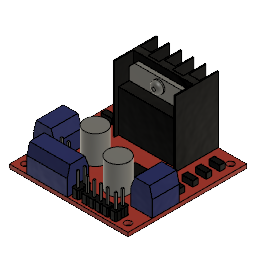
L298n H-Bridge (Autodesk Fusion 360 design; units mm, degrees)
Autodesk Fusion 360 part; units mm, degrees
note: some values were not read from the file. Chosen so that the rebuilt part matches the saved one: which bodies a step acts on; which face or edge a step refers to. Set by a fixed rule: which sketch regions a step uses.
sketch "Sketch1" plane through (0, 0, 0) normal (0, 0, 1) x (1, 0, 0)
  line L0 (0, 0) -> (-70, 0) construction
  line L1 (22, 22) -> (22, -22)
  line L2 (22, -22) -> (-22, -22)
  line L3 (-22, -22) -> (-22, 22)
  line L4 (22, -13) -> (-22, -13) construction
  line L5 (-22, -14) -> (22, -14) construction
  line L6 (-15.5, -22) -> (-15.5, -14) construction
  line L7 (-15.5, -22) -> (-0.5, -22)
  line L8 (-0.5, -22) -> (-0.5, -14)
  line L9 (-0.5, -14) -> (-15.5, -14)
  line L10 (-15.5, -14) -> (-15.5, -22)
  line L11 (-22, -13) -> (-14, -13)
  line L12 (-14, -13) -> (-14, -3)
  line L13 (-14, -3) -> (-22, -3)
  line L14 (-22, -3) -> (-22, -13)
  line L15 (22, -13) -> (14, -13)
  line L16 (14, -13) -> (14, -3)
  line L17 (14, -3) -> (22, -3)
  line L18 (22, -3) -> (22, -13)
  line L19 (-12, 22) -> (-12, 0) construction
  line L20 (12, 22) -> (12, 0) construction
  line L21 (11, 22) -> (11.5, 22)
  line L22 (0, 22) -> (-11.5, 22)
  line L23 (-11.5, 22) -> (-11.5, 6)
  line L24 (11.5, 6) -> (11.5, 22)
  line L25 (-11.5, 22) -> (-11.5, 6)
  line L26 (0, -22) -> (2.5, -22) construction
  line L27 (0, -22) -> (0, -21) construction
  line L28 (0.5, -21) -> (2, -21)
  line L29 (2.5, -18) -> (2.5, -16.5)
  line L30 (2, -16) -> (0.5, -16)
  line L31 (0, -19) -> (0, -20.5)
  line L32 (2.5, -21) -> (3.5, -21) construction
  line L33 (4, -21) -> (5.5388, -21)
  line L34 (13.5, -20.5) -> (13.5, -18.9999)
  line L35 (7.9986, -18.5) -> (6.5388, -18.5)
  line L36 (3.5, -19) -> (3.5, -20.5)
  line L37 (13.5, -21) -> (14, -21) construction
  line L38 (14.5, -21) -> (16, -21)
  line L39 (16.5, -18) -> (16.5, -16.5)
  line L40 (16, -16) -> (14.5, -16)
  line L41 (14, -19) -> (14, -20.5)
  line L42 (-14, -14) -> (-14, -13.5) construction
  line L43 (-14, -13.5) -> (-13.5, -13.5) construction
  line L44 (-10.5, -13.5) -> (-9, -13.5)
  line L45 (-8.5, -13) -> (-8.5, -11.5)
  line L46 (-11.5, -11) -> (-13, -11)
  line L47 (-13.5, -11.5) -> (-13.5, -13)
  line L48 (1.25, -21) -> (1.25, -16) construction
  line L49 (0.5, -18.5) -> (2, -18.5)
  line L50 (3.5, -19.75) -> (13.5, -19.75) construction
  line L51 (8.4986, -19) -> (8.4986, -20.5)
  line L52 (4, -18.5) -> (5.5388, -18.5)
  line L53 (6.0388, -19) -> (6.0388, -20.5)
  line L54 (8.9986, -18.5) -> (10.5014, -18.5)
  line L55 (11.0014, -18.9999) -> (11.0014, -20.5)
  line L56 (14.5, -18.5) -> (16, -18.5)
  arc A0 (0.5, -18.5) -> (0, -19) centre (0.5, -19) ccw
  line L57 (0, -16.5) -> (0, -18)
  arc A1 (0, -18) -> (0.5, -18.5) centre (0.5, -18) ccw
  arc A2 (2, -18.5) -> (2.5, -18) centre (2, -18) ccw
  line L58 (2.5, -20.5) -> (2.5, -19)
  arc A3 (2.5, -19) -> (2, -18.5) centre (2, -19) ccw
  arc A4 (0.5, -16) -> (0, -16.5) centre (0.5, -16.5) ccw
  arc A5 (2.5, -16.5) -> (2, -16) centre (2, -16.5) ccw
  arc A6 (0, -20.5) -> (0.5, -21) centre (0.5, -20.5) ccw
  arc A7 (2, -21) -> (2.5, -20.5) centre (2, -20.5) ccw
  arc A8 (6.5388, -18.5) -> (6.0388, -19) centre (6.5388, -19) ccw
  arc A9 (5.5388, -21) -> (6.0388, -20.5) centre (5.5388, -20.5) ccw
  line L59 (6.5388, -21) -> (7.9986, -21)
  line L60 (8.9986, -21) -> (10.5014, -21)
  line L61 (11.5014, -21) -> (13, -21)
  arc A10 (6.0388, -20.5) -> (6.5388, -21) centre (6.5388, -20.5) ccw
  arc A11 (8.4986, -19) -> (7.9986, -18.5) centre (7.9986, -19) ccw
  arc A12 (7.9986, -21) -> (8.4986, -20.5) centre (7.9986, -20.5) ccw
  arc A13 (3.5, -20.5) -> (4, -21) centre (4, -20.5) ccw
  arc A14 (4, -18.5) -> (3.5, -19) centre (4, -19) ccw
  arc A15 (8.9986, -18.5) -> (8.4986, -19) centre (8.9986, -19) ccw
  arc A16 (8.4986, -20.5) -> (8.9986, -21) centre (8.9986, -20.5) ccw
  arc A17 (11.0014, -19) -> (10.5014, -18.5) centre (10.5014, -19) ccw
  arc A18 (10.5014, -21) -> (11.0014, -20.5) centre (10.5014, -20.5) ccw
  line L62 (13, -18.4999) -> (11.5014, -18.4999)
  arc A19 (11.5014, -18.4999) -> (11.0014, -18.9999) centre (11.5014, -18.9999) ccw
  arc A20 (11.0014, -20.5) -> (11.5014, -21) centre (11.5014, -20.5) ccw
  arc A21 (13, -21) -> (13.5, -20.5) centre (13, -20.5) ccw
  arc A22 (13.5, -18.9999) -> (13, -18.4999) centre (13, -18.9999) ccw
  line L63 (-11, -13) -> (-11, -11.5)
  arc A23 (-11, -11.5) -> (-11.5, -11) centre (-11.5, -11.5) ccw
  line L64 (-9, -11) -> (-10.5, -11)
  arc A24 (-10.5, -11) -> (-11, -11.5) centre (-10.5, -11.5) ccw
  arc A25 (-11, -13) -> (-10.5, -13.5) centre (-10.5, -13) ccw
  line L65 (-13, -13.5) -> (-11.5, -13.5)
  arc A26 (-11.5, -13.5) -> (-11, -13) centre (-11.5, -13) ccw
  arc A27 (-13, -11) -> (-13.5, -11.5) centre (-13, -11.5) ccw
  arc A28 (-13.5, -13) -> (-13, -13.5) centre (-13, -13) ccw
  arc A29 (-8.5, -11.5) -> (-9, -11) centre (-9, -11.5) ccw
  arc A30 (-9, -13.5) -> (-8.5, -13) centre (-9, -13) ccw
  line L66 (-13.5, -12.25) -> (-11, -12.25) construction
  line L67 (-11, -12.25) -> (-8.5, -12.25) construction
  arc A31 (14.5, -16) -> (14, -16.5) centre (14.5, -16.5) ccw
  arc A32 (16.5, -16.5) -> (16, -16) centre (16, -16.5) ccw
  arc A33 (14, -20.5) -> (14.5, -21) centre (14.5, -20.5) ccw
  arc A34 (16, -21) -> (16.5, -20.5) centre (16, -20.5) ccw
  arc A35 (16, -18.5) -> (16.5, -18) centre (16, -18) ccw
  line L68 (16.5, -20.5) -> (16.5, -19)
  arc A36 (16.5, -19) -> (16, -18.5) centre (16, -19) ccw
  arc A37 (14.5, -18.5) -> (14, -19) centre (14.5, -19) ccw
  line L69 (14, -16.5) -> (14, -18)
  arc A38 (14, -18) -> (14.5, -18.5) centre (14.5, -18) ccw
  line L70 (15.25, -18.5) -> (15.25, -16) construction
  line L71 (15.25, -18.5) -> (15.25, -21) construction
  line L72 (12.2507, -21) -> (12.2507, -18.4999) construction
  line L73 (9.75, -21) -> (9.75, -18.5) construction
  line L74 (7.2687, -21) -> (7.2687, -18.5) construction
  arc A39 (6.0388, -19) -> (5.5388, -18.5) centre (5.5388, -19) ccw
  line L75 (4.7694, -21) -> (4.7694, -18.5) construction
  line L76 (0, -19.75) -> (2.5, -19.75) construction
  line L77 (0, -17.25) -> (2.5, -17.25) construction
  line L78 (-12.25, -11) -> (-12.25, -13.5) construction
  line L79 (-9.75, -11) -> (-9.75, -13.5) construction
  line L80 (6.0388, -19) -> (6.0388, 0) construction
  line L81 (14, -8) -> (22, -8) construction
  line L82 (14, -8) -> (14, -13)
  line L83 (14.0388, -9.6848) -> (6.0388, -9.6848) construction
  circle A40 centre (6.0388, -9.6848) radius 4
  line L84 (-8, -14) -> (-8, 3) construction
  line L85 (-14, -4.089) -> (-6, -4.089) construction
  circle A41 centre (-8, -4.089) radius 4
  line L86 (0, 22) -> (0, 15.5)
  line L87 (11.5, 14) -> (11.5, 13)
  line L88 (11, 13) -> (-11, 13)
  line L89 (11.5, 14) -> (11.5, 10.5)
  line L90 (11, 10.5) -> (-11, 10.5)
  line L91 (11.5, 14) -> (11.5, 8.5)
  line L92 (11.5, 6) -> (11, 6)
  line L93 (11, 6) -> (11, 13)
  line L94 (-11.5, 6) -> (-11, 6)
  line L95 (-11, 6) -> (-11, 13)
  line L96 (-11.5, 22) -> (-11, 22)
  line L97 (-11, 22) -> (-11, 15.5)
  line L98 (-11, 22) -> (-7, 22)
  line L99 (-7, 22) -> (-7, 15.5)
  line L100 (-6.5, 14) -> (-6.5, 22)
  line L101 (-6.5, 22) -> (-2.5, 22)
  line L102 (-2.5, 22) -> (-2.5, 14)
  line L103 (-2, 15.5) -> (-2, 22)
  line L104 (11.5, 22) -> (11, 22)
  line L105 (11, 15.5) -> (11, 22)
  line L106 (-22, 22) -> (0, 22)
  line L107 (11, 22) -> (22, 22)
  line L108 (11, 22) -> (0, 22)
  line L109 (11, 22) -> (7, 22)
  line L110 (7, 22) -> (7, 15.5)
  line L111 (6.5, 14) -> (6.5, 22)
  line L112 (6.5, 22) -> (2.5, 22)
  line L113 (2.5, 22) -> (2.5, 14)
  line L114 (2.5, 22) -> (2, 22)
  line L115 (2, 22) -> (2, 15.5)
  line L116 (0, 15.5) -> (-2.5, 15.5)
  line L117 (-7, 15.5) -> (-11, 15.5)
  line L118 (-2.5, 14) -> (-6.5, 14)
  line L119 (0, 0) -> (0, 13) construction
  line L120 (0, 15.5) -> (0, 73.8708) construction
  line L121 (0, 15.5) -> (2, 15.5)
  line L122 (7, 15.5) -> (11, 15.5)
  line L123 (2.5, 14) -> (6.5, 14)
  line L124 (6.5, 14) -> (2.5, 14)
  line L125 (-22, 22) -> (-19, 22) construction
  line L126 (-19, 22) -> (-19, 19) construction
  line L127 (-19, 19) -> (-22, 19) construction
  line L128 (-22, 19) -> (-22, 22) construction
  line L129 (22, 22) -> (19, 22) construction
  line L130 (19, 22) -> (19, 19) construction
  line L131 (19, 19) -> (22, 19) construction
  line L132 (22, 19) -> (22, 22) construction
  line L133 (-22, -22) -> (-19, -22) construction
  line L134 (-19, -22) -> (-19, -19) construction
  line L135 (-19, -19) -> (-22, -19) construction
  line L136 (-22, -19) -> (-22, -22) construction
  line L137 (22, -22) -> (19, -22) construction
  line L138 (19, -22) -> (19, -19) construction
  line L139 (19, -19) -> (22, -19) construction
  line L140 (22, -19) -> (22, -22) construction
  circle A42 centre (19, 19) radius 1.25
  circle A43 centre (19, -19) radius 1.25
  circle A44 centre (-19, -19) radius 1.25
  circle A45 centre (-19, 19) radius 1.25
  line L141 (-22, 22) -> (-17.5, 22)
  line L142 (-17.5, 22) -> (-17.5, 0) construction
  line L143 (-22, -3) -> (-22, -0.5)
  line L144 (-17.5, 0) -> (-17.5, -0.5)
  line L145 (-17.5, -0.5) -> (-19.5, -0.5)
  line L146 (-19.5, -0.5) -> (-15.5, -0.5)
  line L147 (-15.5, -0.5) -> (-15.5, 1.5)
  line L148 (-15.5, 1.5) -> (-19.5, 1.5)
  line L149 (-19.5, 1.5) -> (-19.5, -0.5)
  line L150 (-15.5, 4.5) -> (-15.5, 6.5)
  line L151 (-15.5, 6.5) -> (-19.5, 6.5)
  line L152 (-19.5, 4.5) -> (-15.5, 4.5)
  line L153 (-19.5, 6.5) -> (-19.5, 4.5)
  line L154 (-15.5, 9.5) -> (-15.5, 11.5)
  line L155 (-15.5, 11.5) -> (-19.5, 11.5)
  line L156 (-19.5, 9.5) -> (-15.5, 9.5)
  line L157 (-19.5, 11.5) -> (-19.5, 9.5)
  line L158 (-15.5, 14.5) -> (-15.5, 16.5)
  line L159 (-15.5, 16.5) -> (-19.5, 16.5)
  line L160 (-19.5, 14.5) -> (-15.5, 14.5)
  line L161 (-19.5, 16.5) -> (-19.5, 14.5)
  line L162 (15.5, 14.5) -> (15.5, 16.5)
  line L163 (15.5, 16.5) -> (19.5, 16.5)
  line L164 (19.5, 16.5) -> (19.5, 14.5)
  line L165 (19.5, 14.5) -> (15.5, 14.5)
  line L166 (15.5, 9.5) -> (15.5, 11.5)
  line L167 (15.5, 11.5) -> (19.5, 11.5)
  line L168 (19.5, 9.5) -> (15.5, 9.5)
  line L169 (19.5, 11.5) -> (19.5, 9.5)
  line L170 (15.5, 4.5) -> (15.5, 6.5)
  line L171 (15.5, 6.5) -> (19.5, 6.5)
  line L172 (19.5, 4.5) -> (15.5, 4.5)
  line L173 (19.5, 6.5) -> (19.5, 4.5)
  line L174 (15.5, -0.5) -> (15.5, 1.5)
  line L175 (15.5, 1.5) -> (19.5, 1.5)
  line L176 (19.5, -0.5) -> (15.5, -0.5)
  line L177 (19.5, 1.5) -> (19.5, -0.5)
  line L178 (6.0388, -5.3245) -> (3.0388, -5.3245)
  line L179 (6.0388, -5.3245) -> (9.0388, -5.3245)
  line L180 (9.0388, -5.3245) -> (9.0388, -0.3245)
  line L181 (9.0388, -0.3245) -> (3.0388, -0.3245)
  line L182 (3.0388, -5.3245) -> (3.0388, -0.3245)
  line L183 (9.0388, -5.3245) -> (9.5388, -5.3245)
  line L184 (10.0388, -4.8245) -> (10.0388, -0.8245)
  line L185 (9.0388, -0.3245) -> (9.5388, -0.3245)
  arc A46 (10.0388, -0.8245) -> (9.5388, -0.3245) centre (9.5388, -0.8245) ccw
  arc A47 (9.5388, -5.3245) -> (10.0388, -4.8245) centre (9.5388, -4.8245) ccw
  line L186 (3.0388, -5.124) -> (0.0388, -5.124)
  line L187 (0.0388, -5.124) -> (0.0388, -4.624)
  line L188 (0.0388, -4.624) -> (3.0388, -4.624)
  line L189 (3.0388, -4.624) -> (3.0388, -5.124)
  line L190 (3.0388, -2.8245) -> (4, -2.8245) construction
  line L191 (0.0388, -1.0251) -> (3.0388, -1.0251)
  line L192 (3.0388, -1.0251) -> (3.0388, -0.5251)
  line L193 (0.0388, -0.5251) -> (0.0388, -1.0251)
  line L194 (3.0388, -0.5251) -> (0.0388, -0.5251)
  line L195 (-11, 10.5) -> (-11, 7.5)
  line L196 (-11, 7.5) -> (11, 7.5)
  line L197 (-11.5, 6) -> (-11, 6)
  line L198 (11, 6) -> (11.5, 6)
  line L199 (1.5324, -19.4667) -> (0.9667, -19.4676)
  line L200 (0.9667, -19.4676) -> (0.9676, -20.0333)
  line L201 (0.9676, -20.0333) -> (1.5333, -20.0324)
  line L202 (1.5333, -20.0324) -> (1.5324, -19.4667)
  line L203 (1.5324, -16.9667) -> (0.9667, -16.9676)
  line L204 (0.9667, -16.9676) -> (0.9676, -17.5333)
  line L205 (0.9676, -17.5333) -> (1.5333, -17.5324)
  line L206 (1.5333, -17.5324) -> (1.5324, -16.9667)
  line L207 (5.0547, -19.4696) -> (4.489, -19.4647)
  line L208 (4.489, -19.4647) -> (4.4841, -20.0304)
  line L209 (4.4841, -20.0304) -> (5.0498, -20.0353)
  line L210 (5.0498, -20.0353) -> (5.0547, -19.4696)
  line L211 (7.554, -19.4696) -> (6.9883, -19.4647)
  line L212 (6.9883, -19.4647) -> (6.9834, -20.0304)
  line L213 (6.9834, -20.0304) -> (7.5491, -20.0353)
  line L214 (7.5491, -20.0353) -> (7.554, -19.4696)
  line L215 (10.0353, -19.4696) -> (9.4696, -19.4647)
  line L216 (9.4696, -19.4647) -> (9.4647, -20.0304)
  line L217 (9.4647, -20.0304) -> (10.0304, -20.0353)
  line L218 (10.0304, -20.0353) -> (10.0353, -19.4696)
  line L219 (12.536, -19.4696) -> (11.9704, -19.4646)
  line L220 (11.9704, -19.4646) -> (11.9654, -20.0303)
  line L221 (11.9654, -20.0303) -> (12.531, -20.0353)
  line L222 (12.531, -20.0353) -> (12.536, -19.4696)
  line L223 (15.5353, -19.4696) -> (14.9696, -19.4647)
  line L224 (14.9696, -19.4647) -> (14.9647, -20.0304)
  line L225 (14.9647, -20.0304) -> (15.5304, -20.0353)
  line L226 (15.5304, -20.0353) -> (15.5353, -19.4696)
  line L227 (15.5353, -16.9696) -> (14.9696, -16.9647)
  line L228 (14.9696, -16.9647) -> (14.9647, -17.5304)
  line L229 (14.9647, -17.5304) -> (15.5304, -17.5353)
  line L230 (15.5304, -17.5353) -> (15.5353, -16.9696)
  line L231 (-11.966, -11.9683) -> (-12.5317, -11.966)
  line L232 (-12.5317, -11.966) -> (-12.534, -12.5317)
  line L233 (-12.534, -12.5317) -> (-11.9683, -12.534)
  line L234 (-11.9683, -12.534) -> (-11.966, -11.9683)
  line L235 (-9.4626, -11.9718) -> (-10.0282, -11.9626)
  line L236 (-10.0282, -11.9626) -> (-10.0374, -12.5282)
  line L237 (-10.0374, -12.5282) -> (-9.4718, -12.5374)
  line L238 (-9.4718, -12.5374) -> (-9.4626, -11.9718)
  point P0 (0, -16)
  point P1 (3.5, -18.5)
  point P2 (16.5, -21)
  point P3 (14, -16)
  point P4 (-8.5, -13.5)
  point P5 (-13.5, -11)
  point P6 (10.0388, -5.3245)
  point P7 (1.25, -19.75)
  point P8 (1.25, -19.75)
  point P9 (1.25, -17.25)
  point P10 (4.7694, -19.75)
  point P11 (7.2687, -19.75)
  point P12 (9.75, -19.75)
  point P13 (12.2507, -19.75)
  point P14 (15.25, -19.75)
  point P15 (15.25, -17.25)
  point P16 (-12.25, -12.25)
  point P17 (-9.75, -12.25)
  dimension "d1" = 44
  dimension "d2" = 44
  dimension "d3" = 9
  dimension "d4" = 8
  dimension "d5" = 6.5
  dimension "d6" = 15
  dimension "d7" = 8
  dimension "d8" = 10
  dimension "d9" = 8
  dimension "d10" = 10
  dimension "d11" = 10
  dimension "d12" = 11.5
  dimension "d13" = 11.5
  dimension "d15" = 16
  dimension "d16" = 2.5
  dimension "d17" = 1
  dimension "d18" = 2.5
  dimension "d19" = 5
  dimension "d20" = 1
  dimension "d21" = 10
  dimension "d22" = 2.5
  dimension "d23" = 0.5
  dimension "d24" = 2.5
  dimension "d25" = 5
  dimension "d26" = 5
  dimension "d27" = 2.5
  dimension "d28" = 0.5
  dimension "d29" = 0.5
  dimension "d30" = 0.5
  dimension "d31" = 0.5
  dimension "d32" = 0.5
  dimension "d33" = 0.5
  dimension "d34" = 0.5
  dimension "d35" = 0.5
  dimension "d37" = 0.5
  dimension "d38" = 0.5
  dimension "d39" = 0.5
  dimension "d40" = 0.5
  dimension "d41" = 0.5
  dimension "d42" = 0.5
  dimension "d43" = 0.5
  dimension "d44" = 0.5
  dimension "d45" = 0.5
  dimension "d46" = 0.5
  dimension "d47" = 0.5
  dimension "d48" = 0.5
  dimension "d49" = 0.5
  dimension "d50" = 0.5
  dimension "d51" = 0.5
  dimension "d52" = 0.5
  dimension "d53" = 0.5
  dimension "d54" = 0.5
  dimension "d55" = 0.5
  dimension "d56" = 0.5
  dimension "d57" = 0.5
  dimension "d58" = 0.5
  dimension "d59" = 0.5
  dimension "d60" = 0.5
  dimension "d61" = 0.5
  dimension "d62" = 0.5
  dimension "d63" = 0.5
  dimension "d64" = 0.5
  dimension "d65" = 0.5
  dimension "d66" = 0.5
  dimension "d67" = 0.5
  dimension "d70" = 0.5
  dimension "d79" = 8
  dimension "d80" = 8
  dimension "d82" = 1
  dimension "d83" = 3.5
  dimension "d84" = 5.5
  dimension "d85" = 0.5
  dimension "d86" = 0.5
  dimension "d87" = 4
  dimension "d89" = 4
  dimension "d91" = 4
  dimension "d93" = 4
  dimension "d94" = 2.5
  dimension "d95" = 3
  dimension "d96" = 3
  dimension "d97" = 3
  dimension "d98" = 3
  dimension "d99" = 3
  dimension "d100" = 3
  dimension "d101" = 3
  dimension "d102" = 3
  dimension "d103" = 2.5
  dimension "d104" = 2.5
  dimension "d105" = 2.5
  dimension "d106" = 2.5
  dimension "d107" = 4.5
  dimension "d108" = 2.5
  dimension "d109" = 2
  dimension "d110" = 4
  dimension "d111" = 2
  dimension "d114" = 0
  dimension "d115" = 5
  dimension "d116" = 3
  dimension "d117" = 3
  dimension "d118" = 5
  dimension "d119" = 6
  dimension "d120" = 1
  dimension "d121" = 0.5
  dimension "d122" = 0.5
  dimension "d123" = 3
  dimension "d124" = 0.5
  dimension "d131" = 3
  constraint vertical L119
  constraint perpendicular L0 L119
  constraint horizontal L106
  constraint vertical L1
  constraint horizontal L2
  constraint vertical L3
  constraint symmetric L1 L3 L119
  constraint coincident L3 L4.end
  constraint perpendicular L3 L4
  constraint coincident L1 L5.end
  constraint perpendicular L1 L5
  constraint coincident L5 L6.end
  constraint perpendicular L5 L6
  constraint horizontal L7
  constraint vertical L8
  constraint horizontal L9
  constraint vertical L10
  constraint horizontal L11
  constraint vertical L12
  constraint horizontal L13
  constraint vertical L14
  constraint horizontal L15
  constraint vertical L16
  constraint horizontal L17
  constraint vertical L18
  constraint coincident L0 L19.end
  constraint perpendicular L0 L19
  constraint perpendicular L20 L106
  constraint perpendicular L21 L119
  constraint perpendicular L22 L119
  constraint perpendicular L0 L23
  constraint perpendicular L25 L106
  constraint perpendicular L24 L197
  constraint midpoint L2 L26.start
  constraint perpendicular L8 L26
  constraint perpendicular L2 L27
  constraint horizontal L28
  constraint vertical L29
  constraint horizontal L30
  constraint vertical L31
  constraint perpendicular L29 L32
  constraint horizontal L33
  constraint vertical L34
  constraint horizontal L35
  constraint vertical L36
  constraint perpendicular L34 L37
  constraint horizontal L38
  constraint vertical L39
  constraint horizontal L40
  constraint vertical L41
  constraint perpendicular L5 L42
  constraint perpendicular L42 L43
  constraint horizontal L44
  constraint vertical L45
  constraint horizontal L46
  constraint vertical L47
  constraint perpendicular L33 L53
  constraint perpendicular L33 L55
  constraint coincident P0 L31
  constraint tangent L49 A0
  constraint tangent L31 A0
  constraint perpendicular L30 L57
  constraint coincident L49 A0.start
  constraint tangent L57 A1
  constraint tangent L49 A1
  constraint coincident L32.start L29
  constraint tangent L29 A2
  constraint tangent L49 A2
  constraint perpendicular L28 L58
  constraint coincident L49 A2.start
  constraint tangent L58 A3
  constraint tangent L49 A3
  constraint coincident L30 L48.end
  constraint coincident P0 L57
  constraint coincident P0 L30
  constraint tangent L57 A4
  constraint tangent L30 A4
  constraint tangent L30 A5
  constraint tangent L29 A5
  constraint coincident L28 L48.start
  constraint coincident L27.end L28
  constraint coincident L27.end L31
  constraint tangent L28 A6
  constraint tangent L31 A6
  constraint coincident L32.start L28
  constraint coincident L32.start L58
  constraint tangent L28 A7
  constraint tangent L58 A7
  constraint coincident P1 L35
  constraint tangent L53 A8
  constraint tangent L35 A8
  constraint coincident L37.start L33
  constraint tangent L33 A9
  constraint tangent L53 A9
  constraint perpendicular L51 L59
  constraint coincident L32.end L59
  constraint coincident L53 A9.end
  constraint tangent L59 A10
  constraint tangent L53 A10
  constraint tangent L35 A11
  constraint tangent L51 A11
  constraint tangent L59 A12
  constraint tangent L51 A12
  constraint coincident L36 L50.start
  constraint coincident L32.end L36
  constraint coincident L32.end L33
  constraint tangent L36 A13
  constraint tangent L33 A13
  constraint coincident P1 L36
  constraint coincident P1 L52
  constraint tangent L36 A14
  constraint tangent L52 A14
  constraint coincident L51 A11.start
  constraint tangent L54 A15
  constraint tangent L51 A15
  constraint coincident L51 A12.end
  constraint tangent L51 A16
  constraint tangent L60 A16
  constraint tangent L54 A17
  constraint tangent L55 A17
  constraint tangent L60 A18
  constraint tangent L55 A18
  constraint perpendicular L34 L62
  constraint coincident L55 A17.start
  constraint tangent L55 A19
  constraint tangent L62 A19
  constraint coincident L55 A18.end
  constraint tangent L55 A20
  constraint tangent L61 A20
  constraint coincident L34 L50.end
  constraint coincident L37.start L61
  constraint coincident L37.start L34
  constraint tangent L61 A21
  constraint tangent L34 A21
  constraint tangent L62 A22
  constraint tangent L34 A22
  constraint tangent L46 A23
  constraint tangent L63 A23
  constraint perpendicular L45 L64
  constraint coincident L63 A23.start
  constraint tangent L63 A24
  constraint tangent L64 A24
  constraint coincident L43.end L44
  constraint tangent L63 A25
  constraint tangent L44 A25
  constraint perpendicular L47 L65
  constraint coincident L63 A25.start
  constraint tangent L65 A26
  constraint tangent L63 A26
  constraint coincident P5 L47
  constraint coincident P5 L46
  constraint tangent L47 A27
  constraint tangent L46 A27
  constraint coincident L43.end L47
  constraint coincident L43.end L65
  constraint tangent L47 A28
  constraint tangent L65 A28
  constraint tangent L64 A29
  constraint tangent L45 A29
  constraint coincident P4 L44
  constraint coincident P4 L45
  constraint tangent L44 A30
  constraint tangent L45 A30
  constraint midpoint L47 L66.start
  constraint midpoint L63 L66.end
  constraint perpendicular L63 L66
  constraint midpoint L45 L67.end
  constraint perpendicular L45 L67
  constraint coincident L40 L70.end
  constraint coincident P3 L41
  constraint coincident P3 L40
  constraint tangent L41 A31
  constraint tangent L40 A31
  constraint tangent L40 A32
  constraint tangent L39 A32
  constraint coincident L38 L71.end
  constraint coincident L37.end L41
  constraint coincident L37.end L38
  constraint tangent L41 A33
  constraint tangent L38 A33
  constraint coincident P2 L38
  constraint coincident P2 L39
  constraint tangent L38 A34
  constraint tangent L39 A34
  constraint coincident L39 A34.end
  constraint tangent L56 A35
  constraint tangent L39 A35
  constraint tangent A34 L68
  constraint coincident L56 A35.start
  constraint tangent L56 A36
  constraint tangent L68 A36
  constraint coincident L41 A31.end
  constraint tangent L41 A37
  constraint tangent L56 A37
  constraint tangent A31 L69
  constraint coincident L56 A37.start
  constraint tangent L69 A38
  constraint tangent L56 A38
  constraint midpoint L56 L70.start
  constraint perpendicular L40 L70
  constraint perpendicular L38 L71
  constraint midpoint L61 L72.start
  constraint midpoint L62 L72.end
  constraint perpendicular L62 L72
  constraint midpoint L60 L73.start
  constraint midpoint L54 L73.end
  constraint perpendicular L54 L73
  constraint midpoint L59 L74.start
  constraint midpoint L35 L74.end
  constraint perpendicular L35 L74
  constraint coincident L53 A8.end
  constraint tangent L52 A39
  constraint tangent L53 A39
  constraint midpoint L33 L75.start
  constraint midpoint L52 L75.end
  constraint perpendicular L52 L75
  constraint midpoint L31 L76.start
  constraint midpoint L58 L76.end
  constraint perpendicular L58 L76
  constraint midpoint L57 L77.start
  constraint midpoint L29 L77.end
  constraint midpoint L46 L78.start
  constraint midpoint L65 L78.end
  constraint perpendicular L65 L78
  constraint midpoint L64 L79.start
  constraint midpoint L44 L79.end
  constraint tangent A8 L80
  constraint perpendicular L50 L80
  constraint midpoint L16 L81.start
  constraint midpoint L18 L81.end
  constraint coincident L80 L83.end
  constraint perpendicular L80 L83
  constraint coincident L83.end A40.centre
  constraint midpoint L9 L84.start
  constraint perpendicular L0 L84
  constraint coincident L12 L85.start
  constraint perpendicular L84 L85
  constraint coincident L85 A41.centre
  constraint coincident L84 A41.centre
  constraint perpendicular L86 L197
  constraint midpoint L24 L87.start
  constraint perpendicular L20 L123
  constraint perpendicular L87 L123
  constraint perpendicular L25 L88
  constraint perpendicular L88 L89
  constraint perpendicular L25 L90
  constraint perpendicular L88 L91
  constraint coincident L92.end L197
  constraint perpendicular L88 L93
  constraint perpendicular L23 L94
  constraint perpendicular L88 L95
  constraint coincident L95 L90.end
  constraint coincident L93 L90.start
  constraint coincident L22 L96.end
  constraint perpendicular L97 L98
  constraint perpendicular L100 L106
  constraint coincident L100.end L106
  constraint coincident L101.end L106
  constraint coincident L22 L103.end
  constraint perpendicular L24 L104
  constraint perpendicular L104 L105
  constraint coincident L21.start L106
  constraint collinear L106 L107
  constraint perpendicular L105 L109
  constraint coincident L108 L111.end
  constraint perpendicular L108 L111
  constraint perpendicular L111 L112
  constraint coincident L108 L114.end
  constraint midpoint L88 L119.end
  constraint perpendicular L24 L121
  constraint perpendicular L23 L116
  constraint coincident L102 L116.end
  constraint collinear L116 L117
  constraint collinear L119 L120
  constraint collinear L121 L122
  constraint coincident L116 L103.start
  constraint horizontal L125
  constraint vertical L126
  constraint horizontal L127
  constraint vertical L128
  constraint horizontal L129
  constraint vertical L130
  constraint horizontal L131
  constraint vertical L132
  constraint horizontal L133
  constraint vertical L134
  constraint horizontal L135
  constraint vertical L136
  constraint horizontal L137
  constraint vertical L138
  constraint horizontal L139
  constraint vertical L140
  constraint coincident L130.end L131.start
  constraint coincident L138.end L139.start
  constraint coincident L134.end L135.start
  constraint coincident L126.end L127.start
  constraint perpendicular L126 L141
  constraint perpendicular L141 L142
  constraint perpendicular L0 L143
  constraint perpendicular L144 L145
  constraint parallel L145 L146
  constraint perpendicular L0 L147
  constraint perpendicular L147 L148
  constraint symmetric L119 L145.end L176.start
  constraint symmetric L119 L146.end L174.start
  constraint symmetric L119 L147.end L174.end
  constraint symmetric L119 L148.end L175.end
  constraint symmetric L119 L150.start L170.start
  constraint symmetric L119 L150.end L170.end
  constraint symmetric L119 L151.end L171.end
  constraint symmetric L119 L152.start L172.start
  constraint symmetric L119 L154.start L166.start
  constraint symmetric L119 L154.end L166.end
  constraint symmetric L119 L155.end L167.end
  constraint symmetric L119 L156.start L168.start
  constraint symmetric L119 L158.start L162.start
  constraint symmetric L119 L158.end L162.end
  constraint symmetric L119 L159.end L163.end
  constraint symmetric L119 L160.start L164.end
  constraint coincident L80 L178.start
  constraint perpendicular L80 L178
  constraint perpendicular L80 L179
  constraint perpendicular L179 L180
  constraint perpendicular L180 L181
  constraint perpendicular L180 L183
  constraint perpendicular L183 L184
  constraint perpendicular L184 L185
  constraint tangent L185 A46
  constraint tangent L184 A46
  constraint coincident P6 L183
  constraint coincident P6 L184
  constraint tangent L183 A47
  constraint tangent L184 A47
  constraint horizontal L186
  constraint vertical L187
  constraint horizontal L188
  constraint vertical L189
  constraint coincident L182 L186.start
  constraint midpoint L182 L190.start
  constraint perpendicular L182 L190
  constraint symmetric L186.start L190 L192.end
  constraint symmetric L186.end L190 L193.start
  constraint symmetric L187.end L190 L191.start
  constraint symmetric L188.end L190 L191.end
  constraint perpendicular L90 L195
  constraint coincident L93 L196.end
  constraint perpendicular L93 L196
  constraint collinear L197 L198
  measures "d1" distance of L3.end L1.start
  measures "d2" distance of L3.end L2.end
  measures "d3" distance of L1.end L4.start
  measures "d4" distance of L2.end L5.start
  measures "d5" distance of L2.end L6.start
  measures "d6" distance of L6.start L7.end
  measures "d7" distance of L4.end L11.end
  measures "d8" distance of L4.end L13.end
  measures "d9" distance of L4.start L15.end
  measures "d10" distance of L3.end L19.start
  measures "d11" distance of L1.start L20.start
  measures "d12" distance of L22.start L21.end
  measures "d13" distance of L22.start L22.end
  measures "d15" distance of L22.end L23.end
  measures "d16" distance of L26.start L26.end
  measures "d17" distance of L26.start L27.end
  measures "d18" distance of L27.end L32.start
  measures "d19" distance of L27.end P0
  measures "d20" distance of L32.start L32.end
  measures "d21" distance of L32.end L37.start
  measures "d22" distance of L32.end P1
  measures "d23" distance of L37.start L37.end
  measures "d24" distance of L37.end P2
  measures "d25" distance of L37.end P3
  measures "d26" distance of L43.end P4
  measures "d27" distance of L43.end P5
  measures "d28" radius of A0
  measures "d29" radius of A1
  measures "d30" radius of A2
  measures "d31" radius of A3
  measures "d32" radius of A4
  measures "d33" radius of A5
  measures "d34" radius of A6
  measures "d35" radius of A7
  measures "d37" radius of A8
  measures "d38" radius of A9
  measures "d39" radius of A10
  measures "d40" radius of A11
  measures "d41" radius of A12
  measures "d42" radius of A13
  measures "d43" radius of A14
  measures "d44" radius of A15
  measures "d45" radius of A16
  measures "d46" radius of A17
  measures "d47" radius of A18
  measures "d48" radius of A19
  measures "d49" radius of A20
  measures "d50" radius of A21
  measures "d51" radius of A22
  measures "d52" radius of A23
  measures "d53" radius of A24
  measures "d54" radius of A25
  measures "d55" radius of A26
  measures "d56" radius of A27
  measures "d57" radius of A28
  measures "d58" radius of A29
  measures "d59" radius of A30
  measures "d60" radius of A31
  measures "d61" radius of A32
  measures "d62" radius of A33
  measures "d63" radius of A34
  measures "d64" radius of A35
  measures "d65" radius of A36
  measures "d66" radius of A37
  measures "d67" radius of A38
  measures "d70" radius of A39
  measures "d79" diameter of A40
  measures "d80" diameter of A41
  measures "d82" distance of L87.start L87.end
  measures "d83" distance of L87.start L89.end
  measures "d84" distance of L87.start L91.end
  measures "d85" distance of L24.start L92.end
  measures "d86" distance of L23.end L94.end
  measures "d87" distance of L96.end L98.end
  measures "d89" distance of L100.end L101.end
  measures "d91" distance of L21.start L109.end
  measures "d93" distance of L111.end L112.end
  measures "d94" distance of L119.end L86.end
  measures "d95" distance of L3.end L125.end
  measures "d96" distance of L3.end L127.end
  measures "d97" distance of L1.start L129.end
  measures "d98" distance of L1.start L131.end
  measures "d99" distance of L2.end L133.end
  measures "d100" distance of L2.end L135.end
  measures "d101" distance of L1.end L137.end
  measures "d102" distance of L1.end L139.end
  measures "d103" diameter of A42
  measures "d104" diameter of A43
  measures "d105" diameter of A44
  measures "d106" diameter of A45
  measures "d107" distance of L3.end L141.end
  measures "d108" distance of L13.end L143.end
  measures "d109" distance of L144.end L145.end
  measures "d110" distance of L145.end L146.end
  measures "d111" distance of L146.end L147.end
  measures "d116" distance of L178.start L178.end
  measures "d117" distance of L178.start L179.end
  measures "d118" distance of L179.end L180.end
  measures "d119" distance of L180.end L181.end
  measures "d120" distance of L179.end P6
  measures "d121" radius of A46
  measures "d122" radius of A47
  measures "d123" distance of L186.start L186.end
  measures "d124" distance of L186.start L188.end
  measures "d131" distance of L90.end L195.end
extrude "Extrude1" add sketch "Sketch1" against normal blind 1.5 contours L1 L2 L3 L8 L9 L10 L11 L12 L13 L15 L16 L17 L23 L24 L25 L82 L87 L89 L91 L92 L93 L94 L95 L106 L107 L141 L143 L196 L197 L198 | L1 L15 L16 L17 L18 L82 | L21 L22 L23 L24 L25 L87 L88 L89 L91 L92 L93 L94 L95 L96 L97 L99 L100 L102 L104 L105 L106 L107 L108 L110 L111 L113 L114 L115 L116 L117 L118 L121 L122 L123 L124 L195 L197 L198 | L105 L108 L109 L110 L122 | L2 L7 L8 L9 L10 | L108 L111 L112 L113 L123 L124 | L86 L108 L115 L121 | L3 L11 L12 L13 L14 | L22 L86 L103 L106 L116 | L22 L102 L103 L106 L116 | L90 L93 L95 L195 L196 | L22 L100 L101 L102 L106 L118 | L88 L90 L93 L95 | L22 L97 L98 L99 L106 L117 | L28 L31 L49 A0 L58 A3 A6 A7 | L29 L30 L49 L57 A1 A2 A4 A5 | L33 L36 L52 L53 A9 A13 A14 A39 | L35 L51 L53 A8 L59 A10 A11 A12 | L51 L54 L55 L60 A15 A16 A17 A18 | L34 L55 L61 L62 A19 A20 A21 A22 | L38 L41 L56 A33 A34 L68 A36 A37 | L39 L40 L56 A31 A32 A35 L69 A38 | L44 L45 L63 L64 A24 A25 A29 A30 | L46 L47 L63 A23 L65 A26 A27 A28 | A40 | A41 | L145 L146 L147 L148 L149 | L150 L151 L152 L153 | L154 L155 L156 L157 | L158 L159 L160 L161 | L162 L163 L164 L165 | L166 L167 L168 L169 | L170 L171 L172 L173 | L174 L175 L176 L177 | L178 L179 L180 L181 L182 L189 L192 | L180 L183 L184 L185 A46 A47 | L182 L186 L187 L188 L189 | L182 L191 L192 L193 L194 | L199 L200 L201 L202 | L203 L204 L205 L206 | L207 L208 L209 L210 | L211 L212 L213 L214 | L215 L216 L217 L218 | L219 L220 L221 L222 | L223 L224 L225 L226 | L227 L228 L229 L230 | L231 L232 L233 L234 | L235 L236 L237 L238 makes body 1
extrude "Extrude3" add sketch "Sketch1" along normal blind 22 contours L88 L90 L93 L95 bodies 1
extrude "Extrude4" add sketch "Sketch1" along normal blind 15.5 contours L90 L93 L95 L195 L196 bodies 1
extrude "Extrude5" add sketch "Sketch1" along normal blind 2 contours L145 L146 L147 L148 L149 | L150 L151 L152 L153 | L154 L155 L156 L157 | L158 L159 L160 L161 | L162 L163 L164 L165 | L166 L167 L168 L169 | L170 L171 L172 L173 | L174 L175 L176 L177 bodies 1
extrude "Extrude6" add sketch "Sketch1" along normal blind 2.2 contours L178 L179 L180 L181 L182 L189 L192 bodies 1
extrude "Extrude7" add sketch "Sketch1" along normal blind 1 contours L182 L186 L187 L188 L189 | L182 L191 L192 L193 L194 bodies 1
extrude "Extrude8" add sketch "Sketch1" along normal blind 0.8 contours L180 L183 L184 L185 A46 A47 bodies 1
extrude "Extrude9" add sketch "Sketch1" along normal blind 3 contours L28 L31 L49 A0 L58 A3 A6 A7 | L29 L30 L49 L57 A1 A2 A4 A5 | L33 L36 L52 L53 A9 A13 A14 A39 | L35 L51 L53 A8 L59 A10 A11 A12 | L51 L54 L55 L60 A15 A16 A17 A18 | L34 L55 L61 L62 A19 A20 A21 A22 | L38 L41 L56 A33 A34 L68 A36 A37 | L39 L40 L56 A31 A32 A35 L69 A38 | L44 L45 L63 L64 A24 A25 A29 A30 | L46 L47 L63 A23 L65 A26 A27 A28 | L199 L200 L201 L202 | L203 L204 L205 L206 | L207 L208 L209 L210 | L211 L212 L213 L214 | L215 L216 L217 L218 | L219 L220 L221 L222 | L223 L224 L225 L226 | L227 L228 L229 L230 | L231 L232 L233 L234 | L235 L236 L237 L238 bodies 1
extrude "Extrude10" add sketch "Sketch1" along normal blind 24.5 contours L21 L22 L23 L24 L25 L87 L88 L89 L91 L92 L93 L94 L95 L96 L97 L99 L100 L102 L104 L105 L106 L107 L108 L110 L111 L113 L114 L115 L116 L117 L118 L121 L122 L123 L124 L195 L197 L198 bodies 1
extrude "Extrude12" add sketch "Sketch1" along normal blind 8.5 contours L199 L200 L201 L202 | L203 L204 L205 L206 | L207 L208 L209 L210 | L211 L212 L213 L214 | L215 L216 L217 L218 | L219 L220 L221 L222 | L223 L224 L225 L226 | L227 L228 L229 L230 | L231 L232 L233 L234 | L235 L236 L237 L238 bodies 1
extrude "Extrude13" add sketch "Sketch1" along normal blind 10.5 contours A40 | A41 bodies 1
extrude "Extrude14" add sketch "Sketch1" along normal blind 10 contours L1 L15 L16 L17 L18 L82 | L2 L7 L8 L9 L10 | L3 L11 L12 L13 L14 bodies 1
sketch "Sketch2" plane through (0, 0, 10.5) normal (0, 0, 1) x (-1, 0, 0)
  circle A0 centre (8, 4.089) radius 4
  line L0 (5.84, 7.4557) -> (5.84, 0.7224)
  circle A1 centre (-6.0388, 9.6848) radius 4
  line L1 (-8.2189, 13.0385) -> (-8.2189, 6.3312)
  constraint coincident A0 L0.start
  constraint coincident A0 L0.end
  constraint vertical L0
  constraint coincident A1 L1.start
  constraint coincident A1 L1.end
  constraint vertical L1
chamfer "Chamfer1" distance 1 distance2 4 3 edges at (-8, -22, 10) (22, -8, 10) (-22, -8, 10) measured on face at (-10.5, -16.6667, 10) measured on face at (19.3333, -9.6667, 10) measured on face at (-16.6667, -9.6667, 10) on bodies 1
chamfer "Chamfer2" distance 1.5 distance2 4 3 edges at (-14, -8, 10) (-8, -14, 10) (14, -8, 10) measured on face at (-16.3333, -9.6667, 10) measured on face at (-10.5, -16.3333, 10) measured on face at (18.6667, -9.6667, 10) on bodies 1
sketch "Sketch3" plane through (0, 10.5, 0) normal (0, -1, 0) x (1, 0, 0)
  line L0 (-11, 15.5) -> (11, 15.5)
  line L1 (11, 15.5) -> (11, 22)
  line L2 (11, 22) -> (-11, 22)
  line L3 (-11, 22) -> (-11, 15.5)
  line L4 (-11, 20.1137) -> (-9, 22)
  line L5 (-11, 20.1137) -> (11, 20.1137) construction
  line L6 (-11, 22) -> (-9, 22)
  line L7 (11, 22) -> (9, 22)
  line L8 (9, 22) -> (11, 20.1137)
  line L9 (-11, 19.1384) -> (11, 19.1384) construction
  circle A0 centre (0, 19.1384) radius 2.1688
  dimension "d158" = 2
  constraint coincident L3 L4.start
  constraint coincident L2 L4.end
  constraint coincident L1 L5.end
  constraint perpendicular L1 L5
  constraint coincident L2.end L3.start
  constraint coincident L1.end L2.start
  constraint perpendicular L1 L7
  constraint coincident L3 L9.start
  constraint coincident L1 L9.end
  constraint perpendicular L1 L9
  constraint midpoint L9 A0.centre
  measures "d158" distance of L1.end L7.end
extrude "Extrude15" cut sketch "Sketch3" against normal blind 2.5 contours L2 L3 L4 L6 | L1 L2 L7 L8 bodies 1
extrude "Extrude16" cut 1 faces at (3, 10.5, 17.6667) along direction (0, 1, 0) blind 1 on bodies 1 bodies 1
extrude "Extrude17" add sketch "Sketch3" against normal blind 1 contours A0 bodies 1
extrude "Extrude18" add sketch "Sketch3" along normal blind 1 contours A0 bodies 1
fillet "Fillet1" radius 1.5 1 edges at (-2.022, 9.5, 18.3542) on bodies 1
ref_plane "WorkPlane1" through (0, 0, 0) normal (0, 0, 1) x (1, 0, 0)
split "Split1" by plane through (0, 0, 0) normal (0, 0, 1) bodies 1 makes body 2 at (-4.005, -4.2884, 7) makes body 3 at (-16.6667, -13, 4) makes body 4 at (-11.5, 16.6667, 8.1667) makes body 5 at (16.8333, 11.5, 0.6667) makes body 6 at (-13.178, -12.3439, 3) makes body 7 at (-16.8333, 11.5, 0.6667) makes body 8 at (-5.5, -22, 4) makes body 9 at (-16.8333, 6.5, 0.6667) makes body 10 at (16.6667, -3, 4) makes body 11 at (16.8333, 6.5, 0.6667) makes body 12 at (1.1559, -20.6778, 3) makes body 13 at (16.8333, 16.5, 0.6667) makes body 14 at (15.3435, -20.6784, 3) makes body 15 at (-16.8333, 16.5, 0.6667) makes body 16 at (3.828, -19.8435, 3) makes body 17 at (-16.8333, 1.5, 0.6667) makes body 18 at (5.0388, -3.6579, 2.2) makes body 19 at (16.8333, 1.5, 0.6667) makes body 20 at (10.0338, -9.8842, 7)
ref_plane "WorkPlane2" through (15.25, -18.5, 3) normal (0, 0, 1) x (1, 0, 0)
split "Split2" by plane through (15.25, -18.5, 3) normal (0, 0, 1) bodies 16 12 14 6 makes body 29 at (-12.1546, -11.9675, 4.8333) makes body 30 at (-9.6511, -11.9687, 4.8333) makes body 27 at (15.3467, -19.468, 4.8333) makes body 28 at (15.532, -17.3467, 4.8333) makes body 25 at (1.533, -19.8438, 4.8333) makes body 26 at (1.3438, -16.967, 4.8333) makes body 21 at (9.8467, -19.468, 4.8333) makes body 22 at (12.5327, -19.8467, 4.8333) makes body 23 at (4.8662, -19.468, 4.8333) makes body 24 at (7.3655, -19.468, 4.8333)
extrude "Extrude19" add sketch "Sketch1" along normal blind 24.5 contours L22 L102 L103 L106 L116 bodies 4
